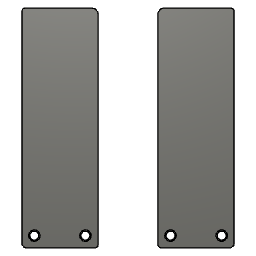
mriya-cnc-mcu-cover (Autodesk Fusion 360 design; units mm, degrees)
Autodesk Fusion 360 part; units mm, degrees
sketch "mriya-mcu-cover" plane through (0, 0, 0) normal (0, 0, 1) x (1, 0, 0)
  circle A0 centre (-22.9, 19.5) radius 1.1
  circle A1 centre (-10.4, 19.5) radius 1.1
  circle A2 centre (-22.9, 19.5) radius 1.4
  circle A3 centre (-10.4, 19.5) radius 1.4
  line L0 (-8.1, 16.5) -> (-24.9, 16.5)
  line L1 (-25.9, 17.5) -> (-25.9, 74.3)
  line L2 (-8.8, 75.1) -> (-25.1, 75.1)
  line L3 (-7.3, 73.6) -> (-7.3, 17.3)
  arc A4 (-7.3, 73.6) -> (-8.8, 75.1) centre (-8.8, 73.6) ccw
  arc A5 (-8.1, 16.5) -> (-7.3, 17.3) centre (-8.1, 17.3) ccw
  arc A6 (-25.1, 75.1) -> (-25.9, 74.3) centre (-25.1, 74.3) ccw
  arc A7 (-25.9, 17.5) -> (-24.9, 16.5) centre (-24.9, 17.5) ccw
  dimension "d8" = 2.2
  dimension "d9" = 2.2
  dimension "d17" = 2.8
  dimension "d18" = 2.8
  constraint concentric A0 A2
  constraint concentric A1 A3
  constraint perpendicular L1 L2
  constraint perpendicular L0 L3
  constraint tangent L2 A4
  constraint tangent L3 A4
  constraint tangent L0 A5
  constraint tangent L3 A5
  constraint tangent L1 A6
  constraint tangent L2 A6
  constraint horizontal L0
  constraint perpendicular L0 L1
  constraint tangent L1 A7
  constraint tangent L0 A7
  measures "d8" diameter of A0
  measures "d9" diameter of A1
  measures "d17" diameter of A2
  measures "d18" diameter of A3
extrude "Extrude5" add sketch "mriya-mcu-cover" along normal blind 1.5 contours L0 L1 L2 L3 A4 A5 A6 A7 makes body 1
extrude "Extrude6" add sketch "mriya-mcu-cover" along normal blind 0.7 contours A2 | A3 bodies 1
mirror "Mirror2" about plane through (0, 0, 0) normal (1, 0, 0) of bodies 1 makes body 2
named bodies: "Left", "Right"
